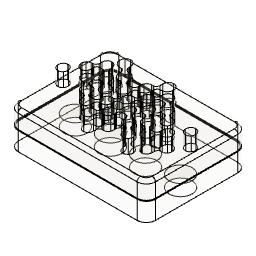
LEDDemov8 (Autodesk Fusion 360 design; units mm, degrees)
Autodesk Fusion 360 part; units mm, degrees
(part 1 of 2)
sketch "Sketch1" plane through (0, 0, 0) normal (0, 0, 1) x (1, 0, 0)
  line L0 (13, -11) -> (-13, -11)
  line L1 (-15, -9) -> (-15, 9)
  line L2 (-13, 11) -> (13, 11)
  line L3 (15, 9) -> (15, -9)
  arc A0 (-13, 11) -> (-15, 9) centre (-13, 9) ccw
  arc A1 (15, 9) -> (13, 11) centre (13, 9) ccw
  arc A2 (-15, -9) -> (-13, -11) centre (-13, -9) ccw
  arc A3 (13, -11) -> (15, -9) centre (13, -9) ccw
  spline S0 degree 3 poles (4.451, 3.5549) (4.7984, 3.5511) (5.0859, 3.2587) (5.1182, 2.8857) knots 0 0 0 0 1 1 1 1
  spline S1 degree 3 poles (5.6944, 1.4602) (5.8606, 1.3558) (6.0486, 1.3007) (6.2391, 1.3007) knots 0 0 0 0 1 1 1 1
  spline S2 degree 2 poles (7.3406, 0.6289) (7.3811, 0.1152) (7.3817, 0.1011) knots 0 0 0 1 1 1
  spline S3 degree 3 poles (8.5391, -0.9433) (8.8097, -0.9225) (9.0589, -0.793) (9.2393, -0.581) knots 0 0 0 0 1 1 1 1
  spline S4 degree 3 poles (9.2393, -0.581) (9.4352, -0.3501) (9.5315, -0.0403) (9.5053, 0.2701) knots 0 0 0 0 1 1 1 1
  spline S5 degree 3 poles (7.991, 1.3352) (7.6348, 1.3467) (7.3433, 1.6295) (7.3137, 1.9883) knots 0 0 0 0 1 1 1 1
  spline S6 degree 3 poles (6.8996, 3.2939) (6.7353, 3.4467) (6.5347, 3.543) (6.3226, 3.5706) knots 0 0 0 0 1 1 1 1
  spline S7 degree 3 poles (6.3226, 3.5706) (6.2485, 3.582) (6.1785, 3.584) (6.0964, 3.5782) knots 0 0 0 0 1 1 1 1
  line L4 (5.0918, 4.2419) -> (5.0454, 4.7799)
  spline S8 degree 3 poles (5.0454, 4.7799) (4.999, 5.3145) (4.603, 5.7508) (4.1055, 5.8168) knots 0 0 0 0 1 1 1 1
  spline S9 degree 3 poles (4.1055, 5.8168) (4.0274, 5.8282) (3.9534, 5.832) (3.8786, 5.8263) knots 0 0 0 0 1 1 1 1
  spline S10 degree 3 poles (2.3232, 3.502) (2.2782, 3.5001) (1.8876, 3.4868) (1.8283, 3.4818) knots 0 0 0 0 1 1 1 1
  spline S11 degree 3 poles (1.8283, 3.4818) (1.5368, 3.4597) (1.2742, 3.3135) (1.0944, 3.0751) knots 0 0 0 0 1 1 1 1
  spline S12 degree 3 poles (1.0944, 3.0751) (0.9578, 2.9041) (0.8742, 2.696) (0.8514, 2.4745) knots 0 0 0 0 1 1 1 1
  line L5 (0.2679, 1.1577) -> (-0.234, 1.1178)
  spline S13 degree 3 poles (-0.234, 1.1178) (-0.7202, 1.0802) (-1.1107, 0.7098) (-1.1827, 0.219) knots 0 0 0 0 1 1 1 1
  spline S14 degree 3 poles (-1.1827, 0.219) (-1.1942, 0.147) (-1.1999, -0.02) (-1.2018, -0.0551) knots 0 0 0 0 1 1 1 1
  line L6 (-1.2018, -0.0551) -> (-1.2132, -0.5365)
  spline S15 degree 3 poles (-3.2654, -2.8819) (-3.2597, -3.2609) (-3.5192, -3.5666) (-3.8694, -3.5935) knots 0 0 0 0 1 1 1 1
  spline S16 degree 2 poles (-3.8694, -3.5935) (-4.1474, -3.605) (-4.7413, -3.6178) knots 0 0 0 1 1 1
  spline S17 degree 3 poles (-4.7413, -3.6178) (-5.0887, -3.6139) (-5.3769, -3.3215) (-5.4099, -2.9384) knots 0 0 0 0 1 1 1 1
  line L7 (-5.4099, -2.9384) -> (-5.4213, -2.7681)
  spline S18 degree 3 poles (-5.4213, -2.7681) (-5.4251, -2.7298) (-5.4227, -2.6717) (-5.4213, -2.6153) knots 0 0 0 0 1 1 1 1
  line L8 (-6.6056, -1.3676) -> (-6.6392, -1.3696)
  spline S19 degree 3 poles (-7.6714, -0.2053) (-7.6707, -0.1939) (-7.6707, -0.1797) (-7.672, -0.1643) knots 0 0 0 0 1 1 1 1
  spline S20 degree 3 poles (-7.672, -0.1643) (-7.7245, 0.4511) (-8.247, 0.9251) (-8.8288, 0.8793) knots 0 0 0 0 1 1 1 1
  spline S21 degree 3 poles (-8.8288, 0.8793) (-9.0995, 0.8585) (-9.3486, 0.7305) (-9.5283, 0.5178) knots 0 0 0 0 1 1 1 1
  spline S22 degree 3 poles (-9.5283, 0.5178) (-9.7243, 0.2875) (-9.8219, -0.0216) (-9.7957, -0.334) knots 0 0 0 0 1 1 1 1
  spline S23 degree 3 poles (-9.7957, -0.334) (-9.7479, -0.8915) (-9.3129, -1.3385) (-8.7817, -1.3756) knots 0 0 0 0 1 1 1 1
  line L9 (-8.7817, -1.3756) -> (-8.2624, -1.3984)
  line L10 (-7.6027, -2.0507) -> (-7.5832, -2.4521)
  spline S24 degree 3 poles (-7.5832, -2.4521) (-7.5813, -2.5006) (-7.5794, -2.5383) (-7.5756, -2.5807) knots 0 0 0 0 1 1 1 1
  spline S25 degree 3 poles (-6.0593, -3.6439) (-5.7045, -3.6554) (-5.4136, -3.9401) (-5.3826, -4.3037) knots 0 0 0 0 1 1 1 1
  line L11 (-5.3827, -4.303) -> (-5.3363, -4.8417)
  spline S26 degree 3 poles (-4.2428, -5.8914) (-4.2185, -5.8914) (-4.1922, -5.8907) (-4.1687, -5.8895) knots 0 0 0 0 1 1 1 1
  spline S27 degree 3 poles (-4.1687, -5.8895) (-3.6415, -5.8477) (-3.2254, -5.3919) (-3.2039, -4.8243) knots 0 0 0 0 1 1 1 1
  line L12 (-3.2039, -4.8243) -> (-3.192, -4.2678)
  spline S28 degree 2 poles (-2.6107, -3.5659) (-2.173, -3.5487) (-2.1185, -3.5443) knots 0 0 0 1 1 1
  spline S29 degree 3 poles (-2.1185, -3.5443) (-1.8283, -3.5222) (-1.5664, -3.3767) (-1.3866, -3.141) knots 0 0 0 0 1 1 1 1
  line L13 (-0.5569, -1.2215) -> (-0.0537, -1.1829)
  spline S30 degree 3 poles (0.908, -0.2916) (0.91, -0.2782) (0.9138, -0.2674) (0.9233, -0.0492) knots 0 0 0 0 1 1 1 1
  line L14 (0.9233, -0.0492) -> (0.9226, 0.4739)
  line L15 (1.5293, 1.1863) -> (1.6329, 1.1939)
  line L16 (1.6329, 1.1939) -> (1.6545, 1.1946)
  spline S31 degree 3 poles (1.6545, 1.1946) (1.6862, 1.1946) (1.7306, 1.1927) (1.7778, 1.1927) knots 0 0 0 0 1 1 1 1
  line L17 (0.091, 5.4475) -> (0.1991, 5.4475)
  line L18 (0.8366, 6.2208) -> (0.8386, 6.8382)
  spline S32 degree 3 poles (0.8386, 6.8373) (0.8462, 7.4897) (1.2943, 8.018) (1.8799, 8.0657) knots 0 0 0 0 1 1 1 1
  spline S33 degree 3 poles (1.8799, 8.0657) (2.5087, 8.1186) (3.0679, 7.585) (3.1251, 6.896) knots 0 0 0 0 1 1 1 1
  spline S34 degree 3 poles (3.1251, 6.896) (3.1327, 6.8101) (3.1308, 6.7229) (3.1213, 6.6377) knots 0 0 0 0 1 1 1 1
  spline S35 degree 3 poles (3.1213, 6.6377) (3.0677, 6.0389) (2.6326, 5.5701) (2.0822, 5.5253) knots 0 0 0 0 1 1 1 1
  line L19 (2.0849, 5.5255) -> (1.548, 5.482)
  spline S36 degree 3 poles (1.548, 5.482) (1.1973, 5.4518) (0.9301, 5.104) (0.9243, 4.6726) knots 0 0 0 0 1 1 1 1
  spline S37 degree 2 poles (0.9243, 4.6726) (0.9281, 4.3064) (0.93, 4.2661) knots 0 0 0 1 1 1
  spline S38 degree 3 poles (0.93, 4.2661) (0.9357, 4.184) (0.9338, 4.0935) (0.9243, 4.0026) knots 0 0 0 0 1 1 1 1
  spline S39 degree 3 poles (0.9243, 4.0026) (0.9016, 3.7582) (0.8105, 3.5256) (0.6638, 3.3341) knots 0 0 0 0 1 1 1 1
  spline S40 degree 3 poles (0.6638, 3.3341) (0.4678, 3.0677) (0.1861, 2.9056) (-0.1287, 2.8799) knots 0 0 0 0 1 1 1 1
  spline S41 degree 3 poles (-0.1287, 2.8799) (-0.1873, 2.8741) (-0.6072, 2.8571) (-0.6556, 2.8543) knots 0 0 0 0 1 1 1 1
  spline S42 degree 3 poles (-0.6556, 2.8543) (-0.999, 2.8272) (-1.2668, 2.4801) (-1.272, 2.0479) knots 0 0 0 0 1 1 1 1
  line L20 (-1.272, 2.0479) -> (-1.2815, 1.4439)
  spline S43 degree 3 poles (-1.2815, 1.4439) (-1.3088, 0.8099) (-1.7548, 0.2992) (-2.3228, 0.253) knots 0 0 0 0 1 1 1 1
  spline S44 degree 3 poles (-2.3228, 0.253) (-2.3491, 0.251) (-2.3764, 0.251) (-2.4035, 0.251) knots 0 0 0 0 1 1 1 1
  spline S45 degree 3 poles (-2.4035, 0.251) (-2.4549, 0.251) (-2.5106, 0.2549) (-2.5673, 0.2644) knots 0 0 0 0 1 1 1 1
  spline S46 degree 3 poles (-2.5673, 0.2644) (-3.1037, 0.3385) (-3.5301, 0.8272) (-3.58, 1.426) knots 0 0 0 0 1 1 1 1
  line L21 (-3.58, 1.426) -> (-3.6285, 2.0292)
  spline S47 degree 3 poles (-3.6284, 2.0285) (-3.6622, 2.4357) (-3.9726, 2.7527) (-4.3505, 2.7681) knots 0 0 0 0 1 1 1 1
  line L22 (-4.3505, 2.7681) -> (-4.669, 2.7739)
  spline S48 degree 3 poles (-4.669, 2.7739) (-4.7102, 2.772) (-4.777, 2.772) (-4.8188, 2.772) knots 0 0 0 0 1 1 1 1
  spline S49 degree 3 poles (-4.8188, 2.772) (-4.8761, 2.772) (-4.9186, 2.7739) (-4.9516, 2.7796) knots 0 0 0 0 1 1 1 1
  spline S50 degree 3 poles (-4.9516, 2.7796) (-5.1769, 2.8119) (-5.3904, 2.9189) (-5.568, 3.09) knots 0 0 0 0 1 1 1 1
  spline S51 degree 3 poles (-5.568, 3.09) (-5.8043, 3.3086) (-5.9511, 3.6183) (-5.979, 3.958) knots 0 0 0 0 1 1 1 1
  spline S52 degree 3 poles (-5.979, 3.958) (-5.9847, 4.0256) (-6.0084, 4.4974) (-6.0097, 4.5517) knots 0 0 0 0 1 1 1 1
  line L23 (-6.7293, 5.3205) -> (-7.288, 5.3478)
  spline S53 degree 3 poles (-7.288, 5.3478) (-7.8611, 5.3881) (-8.3285, 5.8886) (-8.3799, 6.5138) knots 0 0 0 0 1 1 1 1
  spline S54 degree 3 poles (-8.3799, 6.5138) (-8.4078, 6.8683) (-8.3013, 7.2197) (-8.0835, 7.478) knots 0 0 0 0 1 1 1 1
  spline S55 degree 3 poles (-8.0835, 7.478) (-7.8898, 7.7085) (-7.6248, 7.8494) (-7.3394, 7.8728) knots 0 0 0 0 1 1 1 1
  spline S56 degree 3 poles (-7.3394, 7.8728) (-7.3092, 7.8747) (-7.2808, 7.8747) (-7.2514, 7.8747) knots 0 0 0 0 1 1 1 1
  spline S57 degree 3 poles (-7.2514, 7.8747) (-6.6556, 7.8747) (-6.1463, 7.3596) (-6.0927, 6.7014) knots 0 0 0 0 1 1 1 1
  spline S58 degree 2 poles (-6.0927, 6.7014) (-6.092, 6.6802) (-6.0471, 6.1121) knots 0 0 0 1 1 1
  spline S59 degree 3 poles (-6.0471, 6.1121) (-6.0133, 5.6814) (-5.6875, 5.3145) (-5.3169, 5.3108) knots 0 0 0 0 1 1 1 1
  spline S60 degree 3 poles (-4.9354, 5.3146) (-4.9113, 5.3165) (-4.8833, 5.3184) (-4.8539, 5.3184) knots 0 0 0 0 1 1 1 1
  spline S61 degree 3 poles (-4.8539, 5.3184) (-4.6483, 5.3184) (-4.4451, 5.2575) (-4.2668, 5.1402) knots 0 0 0 0 1 1 1 1
  spline S62 degree 3 poles (-4.2668, 5.1402) (-3.9256, 4.9376) (-3.6981, 4.5575) (-3.6629, 4.1268) knots 0 0 0 0 1 1 1 1
  spline S63 degree 3 poles (-3.6629, 4.1268) (-3.6553, 4.0321) (-3.6476, 3.5933) (-3.6457, 3.5426) knots 0 0 0 0 1 1 1 1
  spline S64 degree 3 poles (-3.6457, 3.5426) (-3.6127, 3.1251) (-3.3074, 2.7986) (-2.9347, 2.7942) knots 0 0 0 0 1 1 1 1
  spline S65 degree 3 poles (-7.1378, 0.846) (-6.9742, 0.7397) (-6.787, 0.6837) (-6.5978, 0.6837) knots 0 0 0 0 1 1 1 1
  spline S66 degree 3 poles (-6.5978, 0.6837) (-6.5701, 0.6837) (-6.5453, 0.6851) (-6.5237, 0.6876) knots 0 0 0 0 1 1 1 1
  spline S67 degree 2 poles (-6.5237, 0.6876) (-6.4894, 0.6882) (-6.1703, 0.6914) knots 0 0 0 1 1 1
  spline S68 degree 3 poles (-6.1703, 0.6914) (-5.8302, 0.6876) (-5.5508, 0.3884) (-5.5185, -0.0048) knots 0 0 0 0 1 1 1 1
  spline S69 degree 2 poles (-5.5185, -0.0048) (-5.4788, -0.5105) (-5.4775, -0.5462) knots 0 0 0 1 1 1
  spline S70 degree 3 poles (-5.4775, -0.5462) (-5.4242, -1.1784) (-4.9132, -1.6673) (-4.3288, -1.6194) knots 0 0 0 0 1 1 1 1
  spline S71 degree 3 poles (-4.3288, -1.6194) (-3.7457, -1.5717) (-3.3168, -1.0128) (-3.3693, -0.3745) knots 0 0 0 0 1 1 1 1
  spline S72 degree 3 poles (-3.3693, -0.3745) (-3.4157, 0.1985) (-3.8454, 0.657) (-4.3739, 0.6947) knots 0 0 0 0 1 1 1 1
  line L24 (-4.3739, 0.6947) -> (-4.8701, 0.719)
  spline S73 degree 3 poles (-5.5334, 1.3896) (-5.5347, 1.4394) (-5.5555, 1.8703) (-5.5603, 1.9316) knots 0 0 0 0 1 1 1 1
  spline S74 degree 3 poles (-5.5603, 1.9316) (-5.5866, 2.2427) (-5.7219, 2.5261) (-5.9387, 2.7274) knots 0 0 0 0 1 1 1 1
  spline S75 degree 3 poles (-5.9387, 2.7274) (-6.1017, 2.8849) (-6.2989, 2.9833) (-6.5063, 3.0123) knots 0 0 0 0 1 1 1 1
  spline S76 degree 3 poles (-6.5063, 3.0123) (-6.5838, 3.0237) (-6.6685, 3.0275) (-6.7325, 3.0218) knots 0 0 0 0 1 1 1 1
  line L25 (-6.7325, 3.0218) -> (-6.7615, 3.0218)
  spline S77 degree 3 poles (-6.7615, 3.0218) (-6.8484, 3.0218) (-7.0584, 3.0232) (-7.0618, 3.0232) knots 0 0 0 0 1 1 1 1
  spline S78 degree 3 poles (-7.0618, 3.0232) (-7.4092, 3.0365) (-7.7775, 3.4245) (-7.8085, 3.7988) knots 0 0 0 0 1 1 1 1
  line L26 (-7.8085, 3.7988) -> (-7.8545, 4.353)
  spline S79 degree 3 poles (-7.8543, 4.3503) (-7.8988, 4.8997) (-8.2926, 5.3488) (-8.7895, 5.4168) knots 0 0 0 0 1 1 1 1
  spline S80 degree 3 poles (-8.7895, 5.4168) (-8.8388, 5.4244) (-8.8873, 5.4264) (-8.9357, 5.4264) knots 0 0 0 0 1 1 1 1
  spline S81 degree 3 poles (-8.9357, 5.4264) (-8.9613, 5.4264) (-8.9869, 5.4264) (-9.0146, 5.4244) knots 0 0 0 0 1 1 1 1
  spline S82 degree 3 poles (-9.0146, 5.4244) (-9.5357, 5.3813) (-9.9484, 4.9134) (-9.972, 4.333) knots 0 0 0 0 1 1 1 1
  line L27 (-9.972, 4.333) -> (-9.9839, 3.7582)
  spline S83 degree 3 poles (-9.9835, 3.7795) (-9.9873, 3.3836) (-10.2339, 3.0658) (-10.549, 3.0396) knots 0 0 0 0 1 1 1 1
  spline S84 degree 3 poles (-10.549, 3.0396) (-10.5922, 3.0382) (-10.9779, 3.0243) (-11.0358, 3.0188) knots 0 0 0 0 1 1 1 1
  spline S85 degree 3 poles (2.5888, -2.9803) (2.9288, -2.9841) (3.2096, -3.2846) (3.2413, -3.6678) knots 0 0 0 0 1 1 1 1
  spline S86 degree 3 poles (3.2413, -3.6678) (3.2426, -3.7136) (3.247, -4.1169) (3.2546, -4.2037) knots 0 0 0 0 1 1 1 1
  spline S87 degree 3 poles (3.2546, -4.2037) (3.2869, -4.5983) (3.497, -4.9477) (3.8088, -5.1335) knots 0 0 0 0 1 1 1 1
  spline S88 degree 3 poles (3.8088, -5.1335) (3.9731, -5.2398) (4.1596, -5.2965) (4.3481, -5.2965) knots 0 0 0 0 1 1 1 1
  spline S89 degree 3 poles (4.3481, -5.2965) (4.3723, -5.2965) (4.4, -5.2958) (4.4214, -5.2946) knots 0 0 0 0 1 1 1 1
  spline S90 degree 2 poles (4.4214, -5.2946) (4.4565, -5.2927) (4.7722, -5.2908) knots 0 0 0 1 1 1
  spline S91 degree 3 poles (4.7722, -5.2908) (5.1115, -5.2927) (5.4347, -5.6227) (5.467, -6.018) knots 0 0 0 0 1 1 1 1
  spline S92 degree 2 poles (5.467, -6.018) (5.508, -6.5391) (5.5094, -6.5593) knots 0 0 0 1 1 1
  spline S93 degree 3 poles (5.5094, -6.5593) (5.5592, -7.1633) (6.0258, -7.6359) (6.5719, -7.6359) knots 0 0 0 0 1 1 1 1
  spline S94 degree 3 poles (6.5719, -7.6359) (6.5982, -7.6359) (6.6251, -7.6346) (6.652, -7.6321) knots 0 0 0 0 1 1 1 1
  spline S95 degree 3 poles (6.652, -7.6321) (6.9153, -7.61) (7.1577, -7.4819) (7.3361, -7.2706) knots 0 0 0 0 1 1 1 1
  spline S96 degree 3 poles (7.3361, -7.2706) (7.5354, -7.0336) (7.6344, -6.711) (7.6075, -6.3859) knots 0 0 0 0 1 1 1 1
  spline S97 degree 3 poles (7.6075, -6.3859) (7.5603, -5.8122) (7.1314, -5.3523) (6.6049, -5.316) knots 0 0 0 0 1 1 1 1
  line L28 (6.6049, -5.316) -> (6.1114, -5.2917)
  spline S98 degree 3 poles (6.1114, -5.2917) (5.7646, -5.2803) (5.4381, -4.9598) (5.4084, -4.5915) knots 0 0 0 0 1 1 1 1
  spline S99 degree 3 poles (5.4084, -4.5915) (5.4065, -4.5417) (5.3849, -4.1094) (5.3802, -4.0468) knots 0 0 0 0 1 1 1 1
  spline S100 degree 3 poles (5.3802, -4.0468) (5.3538, -3.7357) (5.2193, -3.4509) (5.0024, -3.2509) knots 0 0 0 0 1 1 1 1
  spline S101 degree 3 poles (5.0024, -3.2509) (4.8394, -3.0935) (4.6436, -2.9957) (4.4375, -2.9661) knots 0 0 0 0 1 1 1 1
  spline S102 degree 3 poles (4.4375, -2.9661) (4.408, -2.9623) (4.3669, -2.9585) (4.3156, -2.9585) knots 0 0 0 0 1 1 1 1
  spline S103 degree 3 poles (4.3156, -2.9585) (4.2772, -2.9585) (4.2138, -2.9604) (4.1768, -2.9623) knots 0 0 0 0 1 1 1 1
  line L29 (4.1768, -2.9623) -> (3.886, -2.9527)
  spline S104 degree 3 poles (3.886, -2.9527) (3.5385, -2.9394) (3.2537, -2.6484) (3.2234, -2.2754) knots 0 0 0 0 1 1 1 1
  line L30 (3.2234, -2.2754) -> (3.179, -1.7226)
  spline S105 degree 3 poles (3.179, -1.7226) (3.1339, -1.1725) (2.7413, -0.7241) (2.2491, -0.6561) knots 0 0 0 0 1 1 1 1
  spline S106 degree 3 poles (2.2491, -0.6561) (2.1972, -0.6465) (2.1474, -0.6446) (2.0997, -0.6446) knots 0 0 0 0 1 1 1 1
  spline S107 degree 3 poles (2.0997, -0.6446) (2.0741, -0.6446) (2.0491, -0.6453) (2.0243, -0.6466) knots 0 0 0 0 1 1 1 1
  spline S108 degree 3 poles (2.0243, -0.6466) (1.5031, -0.6897) (1.0938, -1.1576) (1.0702, -1.7393) knots 0 0 0 0 1 1 1 1
  line L31 (1.0702, -1.7393) -> (1.0588, -2.2935)
  spline S109 degree 3 poles (1.0588, -2.2935) (1.055, -2.69) (0.809, -3.0085) (0.4932, -3.0341) knots 0 0 0 0 1 1 1 1
  spline S110 degree 3 poles (0.4932, -3.0341) (0.4501, -3.036) (0.0643, -3.0532) (0.0097, -3.0576) knots 0 0 0 0 1 1 1 1
  spline S111 degree 3 poles (0.0097, -3.0576) (-0.2791, -3.0799) (-0.5376, -3.2293) (-0.7174, -3.4737) knots 0 0 0 0 1 1 1 1
  spline S112 degree 3 poles (-0.7174, -3.4737) (-0.8514, -3.6495) (-0.9342, -3.8622) (-0.9564, -4.0871) knots 0 0 0 0 1 1 1 1
  spline S113 degree 3 poles (-0.9564, -4.0871) (-0.966, -4.1707) (-0.9679, -4.2533) (-0.9603, -4.3295) knots 0 0 0 0 1 1 1 1
  spline S114 degree 2 poles (-0.9603, -4.3295) (-0.9589, -4.3657) (-0.9564, -4.7025) knots 0 0 0 1 1 1
  spline S115 degree 3 poles (-0.9564, -4.7025) (-0.9603, -5.0984) (-1.2063, -5.4168) (-1.5281, -5.4438) knots 0 0 0 0 1 1 1 1
  line L32 (-1.5281, -5.4438) -> (-2.0189, -5.4842)
  spline S116 degree 3 poles (-2.0189, -5.4842) (-2.5226, -5.5253) (-2.9232, -5.9562) (-2.9717, -6.5056) knots 0 0 0 0 1 1 1 1
  spline S117 degree 3 poles (-2.9717, -6.5056) (-2.9812, -6.5837) (-2.9812, -6.6633) (-2.9755, -6.742) knots 0 0 0 0 1 1 1 1
  spline S118 degree 3 poles (-2.9755, -6.742) (-2.9236, -7.3749) (-2.4099, -7.863) (-1.8329, -7.8152) knots 0 0 0 0 1 1 1 1
  spline S119 degree 3 poles (-1.8329, -7.8152) (-1.2956, -7.7715) (-0.8842, -7.288) (-0.8775, -6.6888) knots 0 0 0 0 1 1 1 1
  line L33 (-0.8775, -6.6888) -> (-0.8736, -6.1447)
  spline S120 degree 3 poles (-0.8736, -6.1447) (-0.8775, -5.7576) (-0.6259, -5.4438) (-0.2886, -5.4129) knots 0 0 0 0 1 1 1 1
  line L34 (-0.2886, -5.4129) -> (-0.1903, -5.4129)
  spline S121 degree 3 poles (-0.1903, -5.4129) (0.1188, -5.4129) (0.1679, -5.409) (0.1834, -5.409) knots 0 0 0 0 1 1 1 1
  spline S122 degree 3 poles (0.1834, -5.409) (0.5443, -5.3795) (0.8601, -5.1491) (1.023, -4.799) knots 0 0 0 0 1 1 1 1
  spline S123 degree 3 poles (1.023, -4.799) (1.1267, -4.5957) (1.1711, -4.3647) (1.153, -4.1318) knots 0 0 0 0 1 1 1 1
  spline S124 degree 2 poles (1.153, -4.1318) (1.1492, -4.0955) (1.1435, -3.7359) knots 0 0 0 1 1 1
  spline S125 degree 3 poles (1.1435, -3.7359) (1.1397, -3.3474) (1.3933, -3.0323) (1.7333, -3.0047) knots 0 0 0 0 1 1 1 1
  spline S126 degree 2 poles (1.7333, -3.0047) (2.0093, -2.9751) (2.5891, -2.9798) knots 0 0 0 1 1 1
  spline S127 degree 3 poles (8.9432, -3.1695) (9.2832, -3.1426) (9.535, -2.8301) (9.5296, -2.4436) knots 0 0 0 0 1 1 1 1
  spline S128 degree 2 poles (9.5296, -2.4436) (9.522, -2.0828) (9.5201, -2.0484) knots 0 0 0 1 1 1
  spline S129 degree 3 poles (9.5201, -2.0484) (9.501, -1.8188) (9.5464, -1.5892) (9.6501, -1.3865) knots 0 0 0 0 1 1 1 1
  spline S130 degree 3 poles (9.6501, -1.3865) (9.8131, -1.0385) (10.1254, -0.8102) (10.4843, -0.7806) knots 0 0 0 0 1 1 1 1
  spline S131 degree 3 poles (10.4843, -0.7806) (11.06, -0.7342) (11.571, -1.2189) (11.6215, -1.8491) knots 0 0 0 0 1 1 1 1
  spline S132 degree 3 poles (11.6215, -1.8491) (11.6292, -1.9306) (11.6253, -2.01) (11.6177, -2.0868) knots 0 0 0 0 1 1 1 1
  spline S133 degree 3 poles (11.6177, -2.0868) (11.5969, -2.3117) (11.5146, -2.5258) (11.3807, -2.7009) knots 0 0 0 0 1 1 1 1
  spline S134 degree 3 poles (11.3807, -2.7009) (11.2023, -2.9459) (10.9444, -3.0947) (10.6582, -3.119) knots 0 0 0 0 1 1 1 1
  spline S135 degree 3 poles (10.6582, -3.119) (10.6004, -3.1228) (10.2186, -3.1384) (10.1748, -3.1398) knots 0 0 0 0 1 1 1 1
  spline S136 degree 3 poles (10.1748, -3.1398) (9.8624, -3.1653) (9.6193, -3.4818) (9.6153, -3.8757) knots 0 0 0 0 1 1 1 1
  line L35 (9.6153, -3.8757) -> (9.6039, -4.4264)
  spline S137 degree 3 poles (9.6039, -4.4264) (9.5809, -5.0048) (9.173, -5.4701) (8.6558, -5.5118) knots 0 0 0 0 1 1 1 1
  spline S138 degree 3 poles (8.6558, -5.5118) (8.6303, -5.5137) (8.6047, -5.5156) (8.5783, -5.5156) knots 0 0 0 0 1 1 1 1
  spline S139 degree 3 poles (8.5783, -5.5156) (8.532, -5.5156) (8.4827, -5.5118) (8.4337, -5.5061) knots 0 0 0 0 1 1 1 1
  spline S140 degree 3 poles (8.4337, -5.5061) (7.9435, -5.4387) (7.5523, -4.9916) (7.5065, -4.4449) knots 0 0 0 0 1 1 1 1
  line L36 (7.5065, -4.4449) -> (7.462, -3.8961)
  spline S141 degree 3 poles (7.462, -3.8961) (7.4317, -3.5238) (7.0655, -3.1373) (6.7241, -3.1245) knots 0 0 0 0 1 1 1 1
  spline S142 degree 3 poles (6.7241, -3.1245) (6.7203, -3.1245) (6.512, -3.1232) (6.4258, -3.1232) knots 0 0 0 0 1 1 1 1
  line L37 (6.4258, -3.1232) -> (6.3968, -3.1232)
  spline S143 degree 3 poles (6.3968, -3.1232) (6.3334, -3.1289) (6.25, -3.1245) (6.174, -3.1136) knots 0 0 0 0 1 1 1 1
  spline S144 degree 3 poles (6.174, -3.1136) (5.9686, -3.0841) (5.7727, -2.9863) (5.6117, -2.8295) knots 0 0 0 0 1 1 1 1
  spline S145 degree 3 poles (5.6117, -2.8295) (5.3963, -2.6289) (5.2623, -2.3474) (5.2367, -2.0384) knots 0 0 0 0 1 1 1 1
  spline S146 degree 3 poles (5.2367, -2.0384) (5.2329, -1.9779) (5.2111, -1.5475) (5.209, -1.4984) knots 0 0 0 0 1 1 1 1
  spline S147 degree 3 poles (5.209, -1.4984) (5.18, -1.1321) (4.8973, -0.8426) (4.5532, -0.8305) knots 0 0 0 0 1 1 1 1
  line L38 (4.5532, -0.8305) -> (4.0617, -0.8076)
  spline S148 degree 3 poles (4.0617, -0.8076) (3.5385, -0.77) (3.113, -0.312) (3.0686, 0.2569) knots 0 0 0 0 1 1 1 1
  spline S149 degree 3 poles (3.0686, 0.2569) (3.0161, 0.8925) (3.4423, 1.448) (4.0173, 1.4951) knots 0 0 0 0 1 1 1 1
  spline S150 degree 3 poles (4.0173, 1.4951) (4.5963, 1.5428) (5.102, 1.0575) (5.1538, 0.4279) knots 0 0 0 0 1 1 1 1
  spline S151 degree 2 poles (5.1538, 0.4279) (5.1552, 0.393) (5.1943, -0.1101) knots 0 0 0 1 1 1
  spline S152 degree 3 poles (5.1943, -0.1101) (5.2273, -0.5019) (5.5054, -0.8002) (5.8407, -0.8029) knots 0 0 0 0 1 1 1 1
  spline S153 degree 2 poles (5.8407, -0.8029) (6.1565, -0.8016) (6.1908, -0.801) knots 0 0 0 1 1 1
  spline S154 degree 3 poles (6.1908, -0.801) (6.2116, -0.799) (6.2379, -0.7972) (6.2635, -0.7972) knots 0 0 0 0 1 1 1 1
  spline S155 degree 3 poles (6.2635, -0.7972) (6.4507, -0.7972) (6.6359, -0.8537) (6.7995, -0.9588) knots 0 0 0 0 1 1 1 1
  spline S156 degree 3 poles (6.7995, -0.9588) (7.1099, -1.146) (7.3186, -1.4921) (7.3502, -1.884) knots 0 0 0 0 1 1 1 1
  spline S157 degree 3 poles (7.3502, -1.884) (7.3579, -1.9695) (7.3655, -2.3701) (7.3655, -2.4159) knots 0 0 0 0 1 1 1 1
  spline S158 degree 3 poles (7.3655, -2.4159) (7.3978, -2.797) (7.7594, -3.1922) (8.0947, -3.1962) knots 0 0 0 0 1 1 1 1
  spline S159 degree 2 poles (8.0947, -3.1962) (8.7121, -3.1848) (8.9437, -3.1712) knots 0 0 0 1 1 1
  spline S160 degree 3 poles (-13.1308, -2.0839) (-12.8433, -2.061) (-12.5833, -1.9209) (-12.3989, -1.688) knots 0 0 0 0 1 1 1 1
  spline S161 degree 3 poles (-12.3989, -1.688) (-12.2212, -1.4611) (-12.1356, -1.1729) (-12.1605, -0.876) knots 0 0 0 0 1 1 1 1
  spline S162 degree 3 poles (-12.1605, -0.876) (-12.2111, -0.2895) (-12.6864, 0.169) (-13.2425, 0.169) knots 0 0 0 0 1 1 1 1
  spline S163 degree 3 poles (-13.2425, 0.169) (-13.2708, 0.169) (-13.2977, 0.1683) (-13.3233, 0.1652) knots 0 0 0 0 1 1 1 1
  spline S164 degree 3 poles (11.8345, 0.7477) (11.8864, 0.1336) (12.4008, -0.3397) (12.9966, -0.2939) knots 0 0 0 0 1 1 1 1
  spline S165 degree 3 poles (12.9966, -0.2939) (13.2848, -0.2718) (13.5447, -0.1304) (13.7285, 0.102) knots 0 0 0 0 1 1 1 1
  spline S166 degree 3 poles (13.7285, 0.102) (13.9075, 0.3289) (13.9918, 0.6177) (13.9669, 0.9147) knots 0 0 0 0 1 1 1 1
  spline S167 degree 3 poles (13.9669, 0.9147) (13.9184, 1.5004) (13.4424, 1.959) (12.8849, 1.959) knots 0 0 0 0 1 1 1 1
  spline S168 degree 3 poles (12.8849, 1.959) (12.8585, 1.959) (12.8316, 1.9583) (12.8047, 1.9552) knots 0 0 0 0 1 1 1 1
  spline S169 degree 3 poles (12.8047, 1.9552) (12.2162, 1.9093) (11.7819, 1.3674) (11.8345, 0.7473) knots 0 0 0 0 1 1 1 1
  spline S170 degree 3 poles (-6.0097, 4.5517) (-6.0427, 4.9524) (-6.3722, 5.309) (-6.7486, 5.3215) (-6.7487, 5.3215) (-6.7487, 5.3215) (-6.7487, 5.3215) knots 0 0 0 0 1 1 1 1.000003 1.000003 1.000003 1.000003
  spline S171 degree 2 poles (-3.0412, 2.7928) (-2.9879, 2.7935) (-2.9347, 2.7942) (-2.3417, 2.8018) (-2.0027, 2.8205) knots 0 0 0 0.010654 0.010654 1.010654 1.010654 1.010654
  spline S172 degree 3 poles (-2.0317, 2.8189) (-2.0222, 2.8197) (-2.0127, 2.8205) (-2.0032, 2.8213) (-1.6333, 2.852) (-1.3559, 3.1941) (-1.3596, 3.6189) knots 0 0 0 0 0.002863 0.002863 0.002863 1.002863 1.002863 1.002863 1.002863
  spline S173 degree 2 poles (-1.3596, 3.6187) (-1.3596, 3.6188) (-1.3596, 3.6189) (-1.3672, 4.0108) (-1.373, 4.0504) knots 0 0 0 0.000028 0.000028 1.000028 1.000028 1.000028
  spline S174 degree 3 poles (-1.3708, 4.0238) (-1.3715, 4.0327) (-1.3723, 4.0415) (-1.373, 4.0504) (-1.3938, 4.3043) (-1.3444, 4.5553) (-1.2314, 4.7769) knots 0 0 0 0 0.002673 0.002673 0.002673 1.002673 1.002673 1.002673 1.002673
  spline S175 degree 3 poles (-1.2693, 4.6959) (-1.2566, 4.7229) (-1.244, 4.7499) (-1.2314, 4.7769) (-1.0523, 5.1592) (-0.7089, 5.4102) (-0.3163, 5.4417) knots 0 0 0 0 0.008938 0.008938 0.008938 1.008938 1.008938 1.008938 1.008938
  spline S176 degree 3 poles (-0.3177, 5.4416) (-0.3172, 5.4417) (-0.3168, 5.4417) (-0.3163, 5.4417) (-0.2972, 5.4432) (-0.2459, 5.4475) (0.091, 5.4475) knots 0 0 0 0 0.000143 0.000143 0.000143 1.000143 1.000143 1.000143 1.000143
  spline S177 degree 3 poles (0.199, 5.4475) (0.5652, 5.482) (0.8403, 5.8225) (0.8367, 6.2437) (0.8367, 6.2437) (0.8367, 6.2437) (0.8367, 6.2438) knots 0 0 0 0 1 1 1 1.000009 1.000009 1.000009 1.000009
  line L39 (-5.3169, 5.3108) -> (-4.9354, 5.3146)
  spline S178 degree 3 poles (-11.0258, 3.0196) (-11.0291, 3.0193) (-11.0325, 3.0191) (-11.0358, 3.0188) (-11.3267, 2.9951) (-11.5866, 2.8443) (-11.767, 2.5986) knots 0 0 0 0 0.001007 0.001007 0.001007 1.001007 1.001007 1.001007 1.001007
  spline S179 degree 3 poles (-11.7404, 2.6335) (-11.7493, 2.6219) (-11.7582, 2.6102) (-11.767, 2.5986) (-11.9018, 2.4223) (-11.9845, 2.2074) (-12.0054, 1.9812) knots 0 0 0 0 0.004387 0.004387 0.004387 1.004387 1.004387 1.004387 1.004387
  spline S180 degree 3 poles (-4.8345, 0.7178) (-4.8464, 0.7182) (-4.8582, 0.7186) (-4.8701, 0.719) (-5.2169, 0.7304) (-5.5031, 1.0226) (-5.5334, 1.3896) knots 0 0 0 0 0.00357 0.00357 0.00357 1.00357 1.00357 1.00357 1.00357
  spline S181 degree 3 poles (-7.696, 1.7751) (-7.6637, 1.3813) (-7.4536, 1.0338) (-7.1378, 0.846) (-7.1278, 0.8401) (-7.1179, 0.8341) (-7.1079, 0.8282) knots 0 0 0 0 1 1 1 1.003475 1.003475 1.003475 1.003475
  spline S182 degree 3 poles (-7.7112, 2.3098) (-7.7099, 2.2639) (-7.7036, 1.8613) (-7.696, 1.7751) (-7.6954, 1.7693) (-7.6949, 1.7634) (-7.6944, 1.7575) knots 0 0 0 0 1 1 1 1.001776 1.001776 1.001776 1.001776
  spline S183 degree 3 poles (-11.9954, 2.0612) (-11.9987, 2.0345) (-12.0021, 2.0079) (-12.0054, 1.9812) (-12.0149, 1.9051) (-12.0149, 1.8249) (-12.0092, 1.7422) knots 0 0 0 0 0.008057 0.008057 0.008057 1.008057 1.008057 1.008057 1.008057
  spline S184 degree 3 poles (-12.0093, 1.7428) (-12.0093, 1.7426) (-12.0092, 1.7424) (-12.0092, 1.7422) (-11.9573, 1.11) (-11.4416, 0.6225) (-10.8592, 0.6696) knots 0 0 0 0 0.000059 0.000059 0.000059 1.000059 1.000059 1.000059 1.000059
  spline S185 degree 3 poles (-10.8602, 0.6695) (-10.8598, 0.6695) (-10.8595, 0.6696) (-10.8592, 0.6696) (-10.4963, 0.6986) (-10.1805, 0.9288) (-10.0162, 1.2783) knots 0 0 0 0 0.000095 0.000095 0.000095 1.000095 1.000095 1.000095 1.000095
  spline S186 degree 3 poles (-10.0505, 1.211) (-10.0457, 1.2205) (-10.0408, 1.23) (-10.036, 1.2395) (-10.0294, 1.2524) (-10.0228, 1.2654) (-10.0162, 1.2783) (-9.9126, 1.4816) (-9.8681, 1.7126) (-9.8863, 1.9428) knots 0 0 0 0 0.003203 0.003203 0.003203 0.007553 0.007553 0.007553 1.007553 1.007553 1.007553 1.007553
  spline S187 degree 2 poles (-9.883, 1.8837) (-9.8846, 1.9133) (-9.8863, 1.9428) (-9.8882, 1.9772) (-9.8958, 2.3401) knots 0 0 0 0.00592 0.00592 1.00592 1.00592 1.00592
  spline S188 degree 3 poles (-9.8939, 2.1514) (-9.8946, 2.2143) (-9.8952, 2.2772) (-9.8958, 2.3401) (-9.8996, 2.7286) (-9.646, 3.0423) (-9.304, 3.07) knots 0 0 0 0 0.018873 0.018873 0.018873 1.018873 1.018873 1.018873 1.018873
  spline S189 degree 2 poles (-9.3043, 3.07) (-9.3041, 3.07) (-9.304, 3.07) (-8.7997, 3.0963) (-8.4468, 3.0948) knots 0 0 0 0.000031 0.000031 1.000031 1.000031 1.000031
  spline S190 degree 3 poles (-8.5075, 3.0948) (-8.4876, 3.0946) (-8.4677, 3.0944) (-8.4478, 3.0942) (-8.1078, 3.0904) (-7.7429, 2.6929) (-7.7112, 2.3098) knots 0 0 0 0 0.005963 0.005963 0.005963 1.005963 1.005963 1.005963 1.005963
  spline S191 degree 3 poles (-13.2837, 0.1683) (-13.2969, 0.1673) (-13.3101, 0.1662) (-13.3233, 0.1652) (-13.9111, 0.1194) (-14.3467, -0.4226) (-14.2942, -1.0427) knots 0 0 0 0 0.00397 0.00397 0.00397 1.00397 1.00397 1.00397 1.00397
  spline S192 degree 3 poles (-14.295, -1.0332) (-14.2947, -1.0362) (-14.2945, -1.0392) (-14.2942, -1.0423) (-14.2424, -1.6563) (-13.7273, -2.1297) (-13.1308, -2.0839) knots 0 0 0 0 0.000916 0.000916 0.000916 1.000916 1.000916 1.000916 1.000916
  spline S193 degree 3 poles (-7.576, -2.5763) (-7.5758, -2.5778) (-7.5757, -2.5793) (-7.5756, -2.5807) (-7.5493, -2.8864) (-7.4107, -3.1645) (-7.1878, -3.3591) knots 0 0 0 0 0.000442 0.000442 0.000442 1.000442 1.000442 1.000442 1.000442
  spline S194 degree 3 poles (-7.2161, -3.3328) (-7.2066, -3.3416) (-7.1972, -3.3503) (-7.1878, -3.3591) (-7.0242, -3.5106) (-6.8269, -3.6048) (-6.6175, -3.6324) knots 0 0 0 0 0.003861 0.003861 0.003861 1.003861 1.003861 1.003861 1.003861
  spline S195 degree 2 poles (-6.5247, -3.642) (-6.4566, -3.642) (-6.3885, -3.642) (-6.3225, -3.642) (-6.0593, -3.6439) knots 0 0 0 0.01362 0.01362 1.01362 1.01362 1.01362
  spline S196 degree 3 poles (-6.6983, -1.3729) (-6.7865, -1.3725) (-6.8748, -1.372) (-6.963, -1.3715) (-7.3104, -1.3696) (-7.5966, -1.0752) (-7.6309, -0.6901) (-7.6436, -0.5472) (-7.6564, -0.4042) (-7.6691, -0.2613) knots 0 0 0 0 0.026463 0.026463 0.026463 1.026463 1.026463 1.026463 1.069516 1.069516 1.069516 1.069516
  spline S197 degree 3 poles (-2.304, -1.2558) (-2.6797, -1.309) (-2.9854, -1.5245) (-3.1423, -1.845) (-3.1541, -1.8691) (-3.1659, -1.8933) (-3.1777, -1.9174) knots 0 0 0 0 1 1 1 1.008065 1.008065 1.008065 1.008065
  spline S198 degree 3 poles (-1.7801, -1.2444) (-1.8713, -1.2444) (-1.9624, -1.2444) (-2.0535, -1.2444) (-2.1721, -1.2444) (-2.2542, -1.2482) (-2.304, -1.2558) knots 0 0 0 0 0.02734 0.02734 0.02734 1.02734 1.02734 1.02734 1.02734
  spline S199 degree 3 poles (0.8514, 1.8807) (0.8475, 1.4949) (0.5948, 1.1845) (0.2656, 1.1575) (0.2257, 1.1543) (0.1857, 1.151) (0.1458, 1.1478) knots 0 0 0 0 1 1 1 1.012014 1.012014 1.012014 1.012014
  spline S200 degree 3 poles (3.8786, 5.8263) (3.3507, 5.7853) (2.9359, 5.3287) (2.913, 4.7604) (2.9103, 4.6933) (2.9076, 4.6261) (2.9049, 4.559) knots 0 0 0 0 1 1 1 1.020161 1.020161 1.020161 1.020161
  spline S201 degree 3 poles (5.7691, 3.582) (5.4129, 3.5935) (5.1221, 3.8776) (5.0918, 4.2419) (5.0778, 4.4098) (5.0638, 4.5777) (5.0499, 4.7455) knots 0 0 0 0 1 1 1 1.05054 1.05054 1.05054 1.05054
  spline S202 degree 3 poles (6.0964, 3.5782) (6.0284, 3.5782) (5.7718, 3.582) (5.7691, 3.582) (5.7691, 3.582) (5.769, 3.582) (5.769, 3.582) knots 0 0 0 0 1 1 1 1.000013 1.000013 1.000013 1.000013
  spline S203 degree 3 poles (7.3799, 0.1208) (7.3805, 0.1142) (7.3811, 0.1076) (7.3817, 0.1011) (7.4355, -0.5143) (7.9546, -0.9917) (8.5391, -0.9433) knots 0 0 0 0 0.001982 0.001982 0.001982 1.001982 1.001982 1.001982 1.001982
  spline S204 degree 3 poles (5.1335, 2.3652) (5.1658, 1.9814) (5.3773, 1.6427) (5.6944, 1.4602) (5.7071, 1.4529) (5.7198, 1.4456) (5.7326, 1.4383) knots 0 0 0 0 1 1 1 1.004404 1.004404 1.004404 1.004404
  spline S205 degree 3 poles (-4.4185, -5.8766) (-4.4109, -5.8777) (-4.4033, -5.8789) (-4.3956, -5.88) (-4.3432, -5.8876) (-4.2926, -5.8914) (-4.2428, -5.8914) knots 0 0 0 0 0.002307 0.002307 0.002307 1.002307 1.002307 1.002307 1.002307
  spline S206 degree 3 poles (-1.1472, -2.5909) (-1.1451, -2.375) (-1.143, -2.1591) (-1.1408, -1.9432) (-1.137, -1.5574) (-0.8843, -1.247) (-0.5557, -1.2214) knots 0 0 0 0 0.064775 0.064775 0.064775 1.064775 1.064775 1.064775 1.064775
  spline S207 degree 2 poles (3.5767, 3.5312) (3.5768, 3.5312) (3.5768, 3.5312) (4.2588, 3.5575) (4.4494, 3.5541) knots 0 0 0 0.000004 0.000004 1.000004 1.000004 1.000004
  spline S208 degree 3 poles (5.1182, 2.8857) (5.1182, 2.8412) (5.1259, 2.448) (5.1335, 2.3652) (5.1341, 2.3585) (5.1347, 2.3518) (5.1354, 2.3452) knots 0 0 0 0 1 1 1 1.002009 1.002009 1.002009 1.002009
  spline S209 degree 3 poles (0.9228, 0.4361) (0.9228, 0.4487) (0.9227, 0.4613) (0.9226, 0.4739) (0.9207, 0.8524) (1.1798, 1.1594) (1.5293, 1.1863) (1.5612, 1.1888) (1.5932, 1.1912) (1.6251, 1.1937) knots 0 0 0 0 0.003785 0.003785 0.003785 1.003785 1.003785 1.003785 1.013397 1.013397 1.013397 1.013397
  spline S210 degree 3 poles (2.8494, 1.7775) (2.8502, 1.779) (2.8509, 1.7805) (2.8517, 1.7819) (2.946, 1.9623) (2.991, 2.1792) (2.9836, 2.4256) (2.9815, 2.4958) (2.9794, 2.566) (2.9772, 2.6361) knots 0 0 0 0 0.000497 0.000497 0.000497 1.000497 1.000497 1.000497 1.021561 1.021561 1.021561 1.021561
  spline S211 degree 3 poles (1.7778, 1.1927) (1.8654, 1.1889) (1.9576, 1.187) (2.0033, 1.1908) (2.0046, 1.1909) (2.0059, 1.191) (2.0072, 1.1911) knots 0 0 0 0 1 1 1 1.000393 1.000393 1.000393 1.000393
  spline S212 degree 2 poles (2.9722, 2.8188) (2.9722, 2.8188) (2.9722, 2.8188) knots 1 1 1 1.000002 1.000002 1.000002
  spline S213 degree 3 poles (2.9722, 2.8188) (2.9683, 3.1972) (3.2293, 3.5029) (3.5768, 3.5312) knots 0.018263 0.018263 0.018263 0.018263 1.018263 1.018263 1.018263 1.018263
  line L40 (2.9722, 2.8189) -> (2.9772, 2.6361)
  spline S214 degree 3 poles (2.0033, 1.1908) (2.3683, 1.2198) (2.6854, 1.4426) (2.8517, 1.7819) knots 0 0 0 0 1 1 1 1
  spline S215 degree 3 poles (-0.0555, -1.1831) (0.4259, -1.1439) (0.8219, -0.7764) (0.908, -0.2916) knots 0.05542 0.05542 0.05542 0.05542 1.05542 1.05542 1.05542 1.05542
  spline S216 degree 3 poles (-1.3866, -3.141) (-1.2594, -2.9827) (-1.1768, -2.7926) (-1.1472, -2.5909) knots 0 0 0 0 0.921422 0.921422 0.921422 0.921422
  spline S217 degree 3 poles (-3.192, -4.2678) (-3.1795, -3.8909) (-2.9288, -3.591) (-2.6107, -3.5659) knots 0.017783 0.017783 0.017783 0.017783 1.000009 1.000009 1.000009 1.000009
  spline S218 degree 3 poles (-5.3459, -4.7293) (-5.3427, -4.7667) (-5.3395, -4.8042) (-5.3363, -4.8417) (-5.2911, -5.3688) (-4.9059, -5.7999) (-4.4185, -5.8766) knots 0 0 0 0 0.011289 0.011289 0.011289 0.995966 0.995966 0.995966 0.995966
  spline S219 degree 3 poles (-6.6175, -3.6324) (-6.5862, -3.6371) (-6.5556, -3.6402) (-6.5247, -3.642) knots 0 0 0 0 0.411257 0.411257 0.411257 0.411257
  spline S220 degree 3 poles (-8.2624, -1.3984) (-7.9149, -1.4179) (-7.6319, -1.6981) (-7.6027, -2.0508) knots 0.015392 0.015392 0.015392 0.015392 1 1 1 1
  line L41 (-7.6714, -0.2053) -> (-7.6691, -0.2613)
  line L42 (-6.6983, -1.3729) -> (-6.6392, -1.3696)
  spline S221 degree 3 poles (-5.9291, -1.5565) (-5.949, -1.5442) (-5.9689, -1.532) (-5.9888, -1.5197) (-6.1774, -1.4039) (-6.4016, -1.3514) (-6.6056, -1.3676) knots 0 0 0 0 0.007012 0.007012 0.007012 1.007012 1.007012 1.007012 1.007012
  spline S222 degree 3 poles (-5.4232, -2.4269) (-5.4232, -2.4269) (-5.4232, -2.4268) (-5.4232, -2.4267) (-5.4522, -2.0667) (-5.6424, -1.7456) (-5.9291, -1.5565) knots 0 0 0 0 0.000024 0.000024 0.000024 0.936406 0.936406 0.936406 0.936406
  spline S223 degree 3 poles (-5.4213, -2.6471) (-5.4213, -2.6365) (-5.4213, -2.6259) (-5.4213, -2.6153) (-5.4213, -2.5446) (-5.4194, -2.4778) (-5.4232, -2.4267) (-5.4232, -2.4265) (-5.4233, -2.4263) (-5.4233, -2.4261) knots 0 0 0 0 0.003181 0.003181 0.003181 1.003181 1.003181 1.003181 1.003236 1.003236 1.003236 1.003236
  spline S224 degree 2 poles (-3.2793, -2.3901) (-3.2771, -2.4421) (-3.2749, -2.494) (-3.2736, -2.5263) (-3.2654, -2.8819) knots 0 0 0 0.0104 0.0104 1.0104 1.0104 1.0104
  spline S225 degree 3 poles (-3.1777, -1.9172) (-3.2443, -2.0663) (-3.2788, -2.228) (-3.2793, -2.3901) knots 0.119033 0.119033 0.119033 0.119033 0.844844 0.844844 0.844844 0.844844
  spline S226 degree 3 poles (-2.0477, -1.2444) (-2.0496, -1.2444) (-2.0516, -1.2444) (-2.0535, -1.2444) knots 0.98136 0.98136 0.98136 0.98136 1 1 1 1
  spline S227 degree 3 poles (-1.2132, -0.5365) (-1.212, -0.8997) (-1.4525, -1.1972) (-1.7801, -1.2444) knots 0 0 0 0 0.968386 0.968386 0.968386 0.968386
  spline S228 degree 2 poles (0.8442, 2.3268) (0.8459, 2.2852) (0.8475, 2.2436) (0.8489, 2.21) (0.8514, 1.8807) knots 0 0 0 0.008331 0.008331 1.008331 1.008331 1.008331
  spline S229 degree 3 poles (0.8514, 2.4745) (0.8466, 2.4242) (0.8441, 2.3744) (0.8442, 2.3268) knots 0 0 0 0 0.623159 0.623159 0.623159 0.623159
  spline S230 degree 3 poles (2.9016, 4.2238) (2.8978, 3.8393) (2.6437, 3.529) (2.3232, 3.502) knots 0.062631 0.062631 0.062631 0.062631 1.062631 1.062631 1.062631 1.062631
  line L43 (2.9049, 4.559) -> (2.9016, 4.2238)
  spline S231 degree 3 poles (7.2849, 2.5075) (7.2846, 2.5108) (7.2843, 2.5142) (7.2841, 2.5175) (7.2598, 2.8212) (7.1211, 3.0979) (6.8996, 3.2939) knots 0 0 0 0 0.001009 0.001009 0.001009 1.001009 1.001009 1.001009 1.001009
  spline S232 degree 3 poles (7.3137, 1.9883) (7.3118, 2.0339) (7.2913, 2.4206) (7.2849, 2.5075) knots 0 0 0 0 0.955909 0.955909 0.955909 0.955909
  spline S233 degree 3 poles (9.5053, 0.2701) (9.4574, 0.8276) (9.0238, 1.276) (8.4926, 1.3123) knots 0 0 0 0 1 1 1 1
  line L44 (7.991, 1.3352) -> (8.4926, 1.3123)
  spline S234 degree 3 poles (6.6727, 1.3083) (6.6727, 1.3083) (6.6727, 1.3083) (6.6727, 1.3083) knots 0.998804 0.998804 0.998804 0.998804 1 1 1 1
  spline S235 degree 3 poles (6.2391, 1.3007) (6.2654, 1.3007) (6.2916, 1.302) (6.3131, 1.3045) (6.3339, 1.3068) (6.3547, 1.3092) (6.3755, 1.3116) knots 0 0 0 0 1 1 1 1.006273 1.006273 1.006273 1.006273
  spline S236 degree 3 poles (6.3755, 1.3116) (6.4746, 1.3105) (6.5736, 1.3094) (6.6727, 1.3083) (7.0215, 1.3045) (7.307, 1.0127) (7.3406, 0.6289) knots 0.030359 0.030359 0.030359 0.030359 0.060081 0.060081 0.060081 1.060081 1.060081 1.060081 1.060081
  point P0 (-15, -11)
  point P1 (-15, 11)
  point P2 (15, 11)
  point P3 (6.3131, 1.3045)
  point P4 (6.6727, 1.3083)
  point P5 (7.2841, 2.5175)
  point P6 (2.913, 4.7604)
  point P7 (0.8475, 2.2436)
  point P8 (0.2656, 1.1575)
  point P9 (-3.1423, -1.845)
  point P10 (-3.2749, -2.494)
  point P11 (-5.4232, -2.4267)
  point P12 (-5.9888, -1.5197)
  point P13 (-7.6309, -0.6901)
  point P14 (-6.3885, -3.642)
  point P15 (-4.3956, -5.88)
  point P16 (-1.1408, -1.9432)
  point P17 (2.9836, 2.4256)
  point P18 (-2.0032, 2.8213)
  point P19 (0.8367, 6.2437)
  point P20 (-6.7486, 5.3215)
  point P21 (-8.4478, 3.0942)
  point P22 (-14.2942, -1.0423)
  point P23 (-10.036, 1.2395)
  dimension "d1" = 30
  dimension "d2" = 22
  dimension "d3" = 2
  dimension "d4" = 2
  dimension "d5" = 2
  dimension "d6" = 2
  constraint horizontal L0
  constraint perpendicular L0 L1
  constraint parallel L0 L2
  constraint parallel L1 L3
  constraint coincident P1 L1
  constraint coincident P1 L2
  constraint tangent L1 A0
  constraint tangent L2 A0
  constraint coincident P2 L2
  constraint coincident P2 L3
  constraint tangent L2 A1
  constraint tangent L3 A1
  constraint coincident P0 L0
  constraint coincident P0 L1
  constraint tangent L0 A2
  constraint tangent L1 A2
  constraint tangent L0 A3
  constraint tangent L3 A3
  constraint coincident L23.start S170
  constraint coincident P20 L23
  constraint coincident L23 S170.end
  constraint coincident S47 L21.end
  constraint coincident S47.start L21
  constraint coincident S171 S172.start
  constraint coincident S172 S173.start
  constraint coincident S173 S174.start
  constraint coincident S174 S175.start
  constraint coincident S175 S176.start
  constraint coincident L17.end S177
  constraint coincident S177.start L17
  constraint coincident L18.start S177
  constraint coincident P19 L18
  constraint coincident L18 S177.end
  constraint coincident S32 L18.end
  constraint coincident S32.start L18
  constraint coincident S35 L19.start
  constraint coincident S35.end L19
  constraint coincident S82 L27.start
  constraint coincident S82.end L27
  constraint coincident S84 S178.start
  constraint coincident S178 S179.start
  constraint coincident S83 L27.end
  constraint coincident S83.start L27
  constraint coincident S79 L26.end
  constraint coincident S79.start L26
  constraint coincident S72 L24.start
  constraint coincident S72.end L24
  constraint coincident S181 S182.end
  constraint coincident S179 S183.start
  constraint coincident S183 S184.start
  constraint coincident S184 S185.start
  constraint coincident S185 S186.start
  constraint coincident S186 S187.start
  constraint coincident S188 S189.start
  constraint coincident S189 S190.start
  constraint coincident S163 S191.start
  constraint coincident S191 S192.start
  constraint coincident L10.start S220
  constraint coincident S220.end L10
  constraint coincident S25 L11.start
  constraint coincident S25.end L11
  constraint coincident S17 L7.start
  constraint coincident S17.end L7
  constraint coincident S222.start S223
  constraint coincident L5.start S199
  constraint coincident P8 L5
  constraint coincident S201 S202.end
  constraint coincident S204 S208.end
  constraint coincident S206 L13.start
  constraint coincident S206.end L13
  constraint coincident S215.start L13
  constraint coincident S213 L40.start
  constraint coincident S212.start L40
  constraint parallel L8 L42
  constraint coincident S222 S223.end
  constraint coincident S197 S225.start
  constraint coincident S198 S226.start
  measures "d1" distance of P1 P2
  measures "d2" distance of P0 P1
  measures "d3" radius of A0
  measures "d4" radius of A1
  measures "d5" radius of A2
  measures "d6" radius of A3